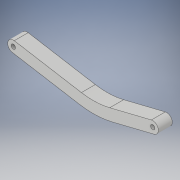
# Autodesk Inventor part: Lever
Saved by Autodesk Inventor 2019.1 (Build 231200000, 200)
## iProperties
Created: 2018-11-01
Part Number: Lever
Material: Generisch
Document SubType Name: Modeling
Designer: JochenAlt
Density: 1 g/cm^3
Appearance: Vorgabe
Author: JochenAlt
Autodesk Inventor part; units mm, degrees
ref_plane "YZ Plane" through (0, 0, 0) normal (1, 0, 0) x (0, 1, 0)
ref_plane "XZ Plane" through (0, 0, 0) normal (0, 1, 0) x (-1, 0, 0)
ref_plane "XY Plane" through (0, 0, 0) normal (0, 0, 1) x (1, 0, 0)
sketch "Skizze1" plane through (0, 0, 0) normal (0, 0, 1) x (1, 0, 0)
  line L0 (0, 0) -> (80, 0) construction
  arc A0 (0.5437, 3.2042) -> (-0.5437, -3.2042) centre (0, 0) ccw
  arc A1 (80.7773, -3.1557) -> (79.2227, 3.1557) centre (80, 0) ccw
  circle A2 centre (0, 0) radius 1.25
  circle A3 centre (80, 0) radius 1.25
  line L1 (0.5437, 3.2042) -> (39.0566, -3.3302)
  line L2 (55.3139, -2.7331) -> (79.2227, 3.1557)
  line L3 (-0.5437, -3.2042) -> (37.9693, -9.7387)
  line L4 (56.8684, -9.0445) -> (80.7773, -3.1557)
  arc A4 (39.0566, -3.3302) -> (55.3139, -2.7331) centre (45.7477, 36.1062) ccw
  arc A5 (37.9693, -9.7387) -> (56.8684, -9.0445) centre (45.7477, 36.1062) ccw
  point P0 (40, 0)
  dimension "d0" = 2.5
  dimension "d1" = 2
  dimension "d2" = 80
  dimension "d6" = 40
  constraints: 12 end point, 8 point on circle, 8 tangent, 6 centre point, 3 coincident, 2 equal radius, 2 parallel, 1 horizontal, 1 midpoint
  measures "d0" diameter of A2
  measures "d1" radial gap between concentric circles of A0 A2
  measures "d2" distance of L0.end L0.start
  measures "d6" radius of A4
extrude "Extrusion1" add sketch "Skizze1" along normal blind 8
